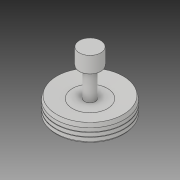
# Autodesk Inventor part: Top1
Saved by Autodesk Inventor 2018 (Build 220112000, 112)
## iProperties
Created: 2017-12-12
Part Number: Top1
Material: Generic
Document SubType Name: Modeling
Designer: Rus
Density: 1 g/cm^3
Appearance: Default
Author: Rus
Autodesk Inventor part; units mm, degrees
ref_plane "YZ Plane" through (0, 0, 0) normal (1, 0, 0) x (0, 1, 0)
ref_plane "XZ Plane" through (0, 0, 0) normal (0, 1, 0) x (-1, 0, 0)
ref_plane "XY Plane" through (0, 0, 0) normal (0, 0, 1) x (1, 0, 0)
sketch "Sketch1" plane through (0, 0, 0) normal (0, 0, 1) x (1, 0, 0)
  line L0 (0, 0) -> (0, 28.575)
  line L1 (0, 0) -> (0, -6.35)
  line L2 (0, 28.575) -> (0, 38.1)
  line L3 (6.35, 28.575) -> (6.35, 38.1)
  line L4 (6.35, 38.1) -> (0, 38.1)
  line L5 (3.175, 17.0324) -> (0, 17.0324) construction
  line L6 (6.35, 28.575) -> (3.175, 28.575)
  line L7 (3.175, 28.575) -> (0, 28.575) construction
  line L8 (0, 0) -> (3.175, 0) construction
  line L9 (3.175, 0) -> (3.175, 0) construction
  line L10 (19.6975, 2.9134) -> (20.32, 3.8024)
  line L11 (0, -6.35) -> (3.175, -4.2333)
  line L12 (3.175, -4.2333) -> (3.175, 0)
  line L13 (3.175, 0) -> (19.6975, 2.9134)
  line L14 (3.175, 28.575) -> (3.175, 11.5094)
  line L15 (20.32, 8.6989) -> (20.1613, 8.5401) construction
  line L16 (20.1613, 8.5401) -> (20.32, 8.3814) construction
  arc A0 (6.35, 38.1) -> (0, 40.0262) centre (0, 28.5962) ccw
  line L17 (20.32, 6.2506) -> (20.1613, 6.0919) construction
  line L18 (20.1613, 6.0919) -> (20.32, 5.9331) construction
  line L19 (20.32, 3.8024) -> (20.32, 5.9331)
  line L20 (20.32, 6.2506) -> (20.32, 8.3814)
  line L21 (20.32, 8.6989) -> (20.32, 10.8296)
  line L22 (20.32, 5.9331) -> (20.32, 6.2506) construction
  line L23 (20.32, 8.3814) -> (20.32, 8.6989) construction
  arc A1 (20.32, 8.6989) -> (20.32, 8.3814) centre (20.4787, 8.5401) ccw
  arc A2 (20.32, 6.2506) -> (20.32, 5.9331) centre (20.4787, 6.0919) ccw
  line L24 (20.1613, 8.5401) -> (0, 8.5401) construction
  line L25 (19.6975, 13.1527) -> (10.3775, 11.5094)
  line L26 (20.32, 10.8296) -> (19.6975, 13.1527)
  line L27 (3.175, 10.2394) -> (3.175, 11.5094) construction
  line L28 (3.175, 11.5094) -> (10.3775, 11.5094)
  line L29 (10.3775, 11.5094) -> (3.175, 10.2394) construction
  line L30 (3.175, 11.5094) -> (3.175, 10.2394) construction
  dimension "d5" = 44.45
  dimension "d6" = 9.525
  dimension "d7" = 6.35
  dimension "d12" = 2.1167
  dimension "d13" = 3.175
  dimension "d15" = 4.2333
  dimension "d24" = 10
  dimension "d28" = 3.175
  dimension "d36" = 0.3175
  dimension "d40" = 11.43
  dimension "d42" = 20.32
  dimension "d43" = 55
  dimension "d46" = 75
  dimension "d47" = 1.27
  dimension "d48" = 10.2394
  dimension "d49" = 0.889
  constraints: 63 end point, 11 vertical, 6 point on circle, 5 equal length, 5 perpendicular, 5 point on line, 4 horizontal, 3 centre point, 2 collinear, 2 parallel, 1 equal radius, 1 line through centre, 1 tangent, 1 vertical alignment
  measures "d5" distance of L2.end L1.end
  measures "d6" distance of L3.start L3.end
  measures "d7" distance between parallel lines of L2 L3
  measures "d12" vertical distance of L11.end L1.end
  measures "d13" horizontal distance of L1.end L11.end
  measures "d15" distance from line of L9 L11.end
  measures "d24" angle of L13 L9
  measures "d28" distance of L3.start L6.end
  measures "d36" distance of L15.start L16.end
  measures "d40" radius of A0
  measures "d42" distance between parallel lines of L20 L0
  measures "d43" angle of L24 L10
  measures "d46" angle of L24 L26
  measures "d47" distance of L27.start L14.end
  measures "d48" distance of L25.start L10.start
  measures "d49" vertical distance of L10.start L10.end
revolve "Revolution1" add sketch "Sketch1" angle 360 about axis through (0, 28.575, 0) along (0, -1, 0)
body "Solid1"
